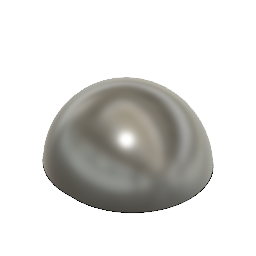
addd (Autodesk Fusion 360 design; units mm, degrees)
Autodesk Fusion 360 part; units mm, degrees
sketch "Sketch1" plane through (0, 0, 0) normal (0, 1, 0) x (1, 0, 0)
  arc A0 (0, 0) -> (0, -65) centre (-2.5, -32.5) ccw
  arc A1 (0, -35) -> (0, -55) centre (-4.0529, -45) ccw
  line L0 (0, 0) -> (0, -35)
  line L1 (0, -55) -> (0, -65)
revolve "Revolve1" add sketch "Sketch1" angle 180 about axis through (0, 0, 0) along (0, 0, -1)
